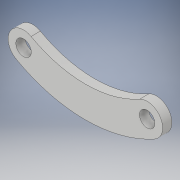
# Autodesk Inventor part: linkageA_mini
Saved by Autodesk Inventor 2017 (Build 210142000, 142)
## iProperties
Created: 2016-08-20
Part Number: linkageA_mini
Material: Generic
Document SubType Name: Modeling
Designer: Nic
Density: 1 g/cm^3
Appearance: Default
Author: Nic
Autodesk Inventor part; units mm, degrees
ref_plane "YZ Plane" through (0, 0, 0) normal (1, 0, 0) x (0, 1, 0)
ref_plane "XZ Plane" through (0, 0, 0) normal (0, 1, 0) x (-1, 0, 0)
ref_plane "XY Plane" through (0, 0, 0) normal (0, 0, 1) x (1, 0, 0)
sketch "Sketch1" plane through (0, 0, 0) normal (0, 0, 1) x (1, 0, 0)
  circle A0 centre (0, 0) radius 1.25
  line L0 (0, 0) -> (20, 0) construction
  circle A1 centre (20, 0) radius 1.25
  arc A2 (1.2195, 2.1824) -> (-1.2195, -2.1824) centre (0, 0) ccw
  arc A3 (21.2195, -2.1824) -> (18.7805, 2.1824) centre (20, 0) ccw
  arc A4 (1.2195, 2.1824) -> (18.7805, 2.1824) centre (10, 17.8955) ccw
  arc A5 (-1.2195, -2.1824) -> (21.2195, -2.1824) centre (10, 17.8955) ccw
  dimension "d0" = 2.5
  dimension "d1" = 20
  dimension "d8" = 5
  dimension "d17" = 18
  constraints: 8 point on circle, 6 centre point, 5 coincident, 3 tangent, 2 end point, 2 equal radius, 1 horizontal
  measures "d0" diameter of A0
  measures "d1" distance of L0.start L0.end
  measures "d8" diameter of A2
  measures "d17" radius of A4
extrude "Extrusion1" add sketch "Sketch1" along normal blind 1.5
body "Solid1"
